Autodesk Fusion 360 part; units mm, degrees
note: some values were not read from the file. Set by a fixed rule: which face or edge a step refers to.
(part 4 of 5)
extrude "Extrude1''''''''''''" add sketch "Sketch1 (10)" along normal blind 5 separate body contours A14 L68 | A14 A15 A16 A17 L68 L69 L70 L71 | A15 L68 | A16 L70 | A17 L70 | L18 L19 L20 L21 picked at (89.8243, -16.6208) picked at (113.8243, -16.6208) picked at (90.3265, -30.2159) picked at (114.3265, -30.2159) makes body 18 in component "R_R_Wheel_Base"
sketch "Sketch2 (11)" plane through (0, -31.65, 0) normal (0, -1, 0) x (1, 0, 0) in component "R_R_Wheel_Base"
  circle A0 centre (115.415, -23.47) radius 1
  circle A1 centre (89.585, -23.47) radius 1
  line L0 (118, -30.47) -> (118, -16.47)
  line L1 (118, -16.47) -> (87, -16.47)
  line L2 (87, -16.47) -> (87, -30.47)
  line L3 (87, -30.47) -> (118, -30.47)
  line L4 (112, -28) -> (93, -28)
  line L5 (93, -28) -> (93, -18.94)
  line L6 (93, -18.94) -> (112, -18.94)
  line L7 (112, -18.94) -> (112, -28)
  line L8 (112, -28) -> (93, -18.94) construction
  line L9 (93, -28) -> (112, -18.94) construction
  point P0 (102.5, -23.47)
  constraint horizontal L4
  constraint perpendicular L4 L5
  constraint parallel L4 L6
  constraint parallel L5 L7
  constraint coincident L8 P0
  constraint coincident L9 P0
extrude "Extrude2''''''''''" add sketch "Sketch2 (11)" along normal blind 16 contours L4 L5 L6 L7 bodies 18 in component "R_R_Wheel_Base"
sketch "Sketch3 (7)" plane through (0, 0, -28) normal (0, 0, -1) x (-1, 0, 0) in component "R_R_Wheel_Base"
  line L0 (-93, -31.65) -> (-112, -31.65)
  line L1 (-112, -31.65) -> (-112, -47.65)
  line L2 (-112, -47.65) -> (-93, -47.65)
  line L3 (-93, -47.65) -> (-93, -31.65)
  line L4 (-93, -39.65) -> (-112, -47.65)
  line L5 (-93, -31.65) -> (-112, -39.65)
  line L6 (-112, -47.65) -> (-135.0409, -57.3514)
  line L7 (-135.0409, -57.3514) -> (-139.3591, -47.0957) construction
  line L8 (-112, -39.65) -> (-137.9021, -50.5561)
  line L9 (-150.0409, -57.3514) -> (-150.0409, -72.3514)
  line L10 (-150.0409, -72.3514) -> (-135.0409, -72.3514)
  line L11 (-135.0409, -72.3514) -> (-135.0409, -57.3514)
  line L12 (-150.0409, -57.3514) -> (-150.0409, -50.5561)
  line L13 (-150.0409, -50.5561) -> (-137.9021, -50.5561)
  line L14 (-135.0409, -57.3514) -> (-150.0409, -57.3514)
  dimension "d472" = 25
  dimension "d473" = 15
  dimension "d474" = 15
  dimension "d476" = 157.166
  dimension "d477" = 6.7953
  constraint midpoint L3 L4.start
  constraint coincident L1.end L2.start
  constraint coincident L0.start L3.end
  constraint midpoint L1 L5.end
  constraint parallel L4 L6
  constraint perpendicular L6 L7
  constraint coincident L7 L8.end
  constraint perpendicular L7 L8
  constraint vertical L9
  constraint horizontal L10
  constraint vertical L11
  constraint perpendicular L12 L13
  measures "d472" distance of L1.end L6.end
  measures "d473" distance of L6.end L9.start
  measures "d474" distance of L6.end L10.end
  measures "d476" angle of L8 L13
  measures "d477" distance of L9.start L12.end
extrude "Extrude4''''''''" add sketch "Sketch3 (7)" against normal blind 20 separate body contours L9 L10 L11 L14 makes body 19 in component "R_R_Wheel_Base"
extrude "Extrude3''''''''" add sketch "Sketch3 (7)" against normal blind 9.06 contours L1 L6 L8 L12 L13 L14 bodies 18 in component "R_R_Wheel_Base"
sketch "Sketch4 (9)" plane through (0, -26.65, 0) normal (0, 1, 0) x (-1, 0, 0) in component "R_R_Wheel_Base"
  circle A0 centre (-115.415, -23.47) radius 1
  circle A1 centre (-89.585, -23.47) radius 1
  line L0 (-118, -16.47) -> (-118, -30.47)
  line L1 (-118, -30.47) -> (-87, -30.47)
  line L2 (-87, -30.47) -> (-87, -16.47)
  line L3 (-87, -16.47) -> (-118, -16.47)
  line L4 (-112.5, -27.97) -> (-92.5, -27.97) construction
  line L5 (-92.5, -27.97) -> (-92.5, -18.97) construction
  line L6 (-92.5, -18.97) -> (-112.5, -18.97) construction
  line L7 (-92.5, -27.97) -> (-112.5, -27.97)
  line L8 (-112.5, -27.97) -> (-112.5, -18.97)
  line L9 (-112.5, -18.97) -> (-92.5, -18.97)
  line L10 (-92.5, -18.97) -> (-92.5, -27.97)
  line L11 (-112.41, -19.06) -> (-92.59, -19.06)
  line L12 (-92.59, -19.06) -> (-92.59, -27.88)
  line L13 (-92.59, -27.88) -> (-112.41, -27.88)
  line L14 (-112.41, -27.88) -> (-112.41, -19.06)
  dimension "d482" = 20
  dimension "d483" = 0.09
  constraint coincident L5.end L6.start
  constraint perpendicular L5 L6
  constraint horizontal L7
  constraint vertical L8
  constraint horizontal L9
  constraint vertical L10
  constraint coincident L4.end L5.start
  measures "d482" distance of L5.end L6.end
extrude "Extrude5'''''" add sketch "Sketch4 (9)" along normal blind 3 contours L11 L12 L13 L14 bodies 18 in component "R_R_Wheel_Base"
sketch "Sketch5 (6)" plane through (0, 0, -28) normal (0, 0, -1) x (-1, 0, 0) in component "R_R_Wheel_Base"
  line L0 (-135.0409, -57.3514) -> (-150.0409, -57.3514)
  line L1 (-150.0409, -57.3514) -> (-150.0409, -72.3514)
  line L2 (-150.0409, -72.3514) -> (-135.0409, -72.3514)
  line L3 (-135.0409, -72.3514) -> (-135.0409, -57.3514)
  line L4 (-136.4409, -69.9514) -> (-148.6409, -69.9514)
  line L5 (-148.6409, -69.9514) -> (-148.6409, -59.7514)
  line L6 (-148.6409, -59.7514) -> (-136.4409, -59.7514)
  line L7 (-136.4409, -59.7514) -> (-136.4409, -69.9514)
  line L8 (-136.4409, -69.9514) -> (-148.6409, -59.7514) construction
  line L9 (-148.6409, -69.9514) -> (-136.4409, -59.7514) construction
  point P0 (-142.5409, -64.8514)
  dimension "d486" = 12.2
  dimension "d487" = 10.2
  constraint horizontal L4
  constraint perpendicular L4 L5
  constraint parallel L4 L6
  constraint parallel L5 L7
  constraint coincident L8 P0
  constraint coincident L9 P0
  measures "d486" distance of L5.end L6.end
  measures "d487" distance of L4.end L5.end
extrude "Extrude6'''''" cut sketch "Sketch5 (6)" against normal blind 18.841 contours L4 L5 L6 L7 bodies 19 in component "R_R_Wheel_Base"
sketch "Sketch6 (6)" plane through (0, 0, -8) normal (0, 0, 1) x (1, 0, 0) in component "R_R_Wheel_Base"
  line L0 (150.0409, -57.3514) -> (135.0409, -57.3514)
  line L1 (135.0409, -57.3514) -> (135.0409, -72.3514)
  line L2 (135.0409, -72.3514) -> (150.0409, -72.3514)
  line L3 (150.0409, -72.3514) -> (150.0409, -57.3514)
  circle A0 centre (142.5409, -64.8514) radius 2
  dimension "d490" = 4
  measures "d490" diameter of A0
extrude "Extrude7''" cut sketch "Sketch6 (6)" against normal blind 1.159 contours A0 bodies 19 in component "R_R_Wheel_Base"
sketch "Sketch7 (4)" plane through (0, 0, -8) normal (0, 0, 1) x (1, 0, 0) in component "R_R_Wheel_Base"
  circle A0 centre (142.5409, -64.8514) radius 2
  line L0 (150.0409, -57.3514) -> (135.0409, -57.3514)
  line L1 (135.0409, -57.3514) -> (135.0409, -72.3514)
  line L2 (135.0409, -72.3514) -> (150.0409, -72.3514)
  line L3 (150.0409, -72.3514) -> (150.0409, -57.3514)
  line L4 (142.5409, -64.8514) -> (137.9689, -64.8514) construction
  line L5 (142.5409, -64.8514) -> (147.1129, -64.8514) construction
  circle A1 centre (137.9689, -64.8514) radius 0.75
  circle A2 centre (147.1129, -64.8514) radius 0.75
  dimension "d493" = 4.572
  dimension "d494" = 4.572
  dimension "d495" = 1.5
  dimension "d496" = 1.5
  constraint coincident A0.centre L4.start
  constraint horizontal L4
  constraint parallel L4 L5
  constraint coincident L4.end A1.centre
  constraint coincident L5.end A2.centre
  measures "d493" distance of A0.centre L4.end
  measures "d494" distance of A0.centre L5.end
  measures "d495" diameter of A1
  measures "d496" diameter of A2
extrude "Extrude8''" cut sketch "Sketch7 (4)" against normal blind 1.159 contours A1 | A2 bodies 19 in component "R_R_Wheel_Base"
sketch "Sketch1 (11)" plane through (0, -26.65, 0) normal (0, -1, 0) x (1, 0, 0) in component "L_R_Wheel_Base"
  line L0 (0, -40) -> (-5, -45)
  line L1 (-5, -45) -> (-5, -79.85)
  line L2 (-5, -79.85) -> (0, -84.85)
  line L3 (0, -84.85) -> (0, -97)
  arc A0 (0, -97) -> (3, -100) centre (3, -97) ccw
  line L4 (3, -100) -> (6, -103)
  line L5 (6, -103) -> (25, -103)
  line L6 (25, -103) -> (28, -100)
  line L7 (28, -100) -> (154, -100)
  arc A1 (154, -100) -> (157, -97) centre (154, -97) ccw
  line L8 (157, -97) -> (157, -94)
  arc A2 (160, -91) -> (157, -94) centre (160, -94) ccw
  line L9 (160, -91) -> (181.27, -91)
  arc A3 (181.27, -91) -> (184.27, -88) centre (181.27, -88) ccw
  line L10 (184.27, -88) -> (184.27, -12)
  arc A4 (184.27, -12) -> (181.27, -9) centre (181.27, -12) ccw
  line L11 (181.27, -9) -> (160, -9)
  arc A5 (157, -6) -> (160, -9) centre (160, -6) ccw
  line L12 (157, -6) -> (157, -3)
  arc A6 (157, -3) -> (154, 0) centre (154, -3) ccw
  line L13 (154, 0) -> (28, 0)
  line L14 (28, 0) -> (25, 3)
  line L15 (25, 3) -> (6, 3)
  line L16 (6, 3) -> (3, 0)
  arc A7 (3, 0) -> (0, -3) centre (3, -3) ccw
  line L17 (0, -3) -> (0, -40)
  circle A8 centre (3, -97) radius 1.0625
  circle A9 centre (3, -71) radius 1.0625
  circle A10 centre (22, -71) radius 1.0625
  circle A11 centre (3, -29) radius 1.0625
  circle A12 centre (3, -3) radius 1.0625
  circle A13 centre (22, -29) radius 1.0625
  circle A14 centre (90, -16) radius 1.0625
  circle A15 centre (114, -16) radius 1.0625
  circle A16 centre (90, -30.28) radius 1.0625
  circle A17 centre (114, -30.28) radius 1.0625
  circle A18 centre (114, -69.72) radius 1.0625
  circle A19 centre (90, -84) radius 1.0625
  circle A20 centre (90, -69.72) radius 1.0625
  circle A21 centre (114, -84) radius 1.0625
  line L18 (92.5, -27.97) -> (92.5, -18.97)
  line L19 (92.5, -18.97) -> (112.5, -18.97)
  line L20 (112.5, -18.97) -> (112.5, -27.97)
  line L21 (112.5, -27.97) -> (92.5, -27.97)
  circle A22 centre (11.5, -70.07) radius 1
  circle A23 centre (11.5, -4.1) radius 1
  circle A24 centre (11.5, -29.93) radius 1
  line L22 (92.5, -81.36) -> (92.5, -72.36)
  line L23 (92.5, -72.36) -> (112.5, -72.36)
  line L24 (112.5, -72.36) -> (112.5, -81.36)
  line L25 (112.5, -81.36) -> (92.5, -81.36)
  circle A25 centre (89.585, -23.47) radius 1
  circle A26 centre (115.415, -76.86) radius 1
  line L26 (16, -72.97) -> (16, -93)
  line L27 (16, -93) -> (7, -93)
  line L28 (7, -93) -> (7, -72.97)
  line L29 (7, -72.97) -> (16, -72.97)
  line L30 (16, -7) -> (16, -27.03)
  line L31 (16, -27.03) -> (7, -27.03)
  line L32 (7, -27.03) -> (7, -7)
  line L33 (7, -7) -> (16, -7)
  circle A27 centre (11.5, -95.9) radius 1
  circle A28 centre (89.585, -76.86) radius 1
  circle A29 centre (115.415, -23.47) radius 1
  line L34 (127.5, -73.5) -> (124.5, -73.5)
  line L35 (124.5, -73.5) -> (124.5, -68.5)
  line L36 (124.5, -68.5) -> (127.5, -68.5)
  line L37 (127.5, -68.5) -> (127.5, -73.5)
  line L38 (183.5, -73.5) -> (180.5, -73.5)
  line L39 (180.5, -73.5) -> (180.5, -68.5)
  line L40 (180.5, -68.5) -> (183.5, -68.5)
  line L41 (183.5, -68.5) -> (183.5, -73.5)
  line L42 (127.5, -31.5) -> (124.5, -31.5)
  line L43 (124.5, -31.5) -> (124.5, -26.5)
  line L44 (124.5, -26.5) -> (127.5, -26.5)
  line L45 (127.5, -26.5) -> (127.5, -31.5)
  line L46 (183.5, -31.5) -> (180.5, -31.5)
  line L47 (180.5, -31.5) -> (180.5, -26.5)
  line L48 (180.5, -26.5) -> (183.5, -26.5)
  line L49 (183.5, -26.5) -> (183.5, -31.5)
  line L50 (36.83, -3.81) -> (36.83, -13.97)
  line L51 (36.83, -13.97) -> (19.05, -13.97)
  line L52 (19.05, -13.97) -> (19.05, -3.81)
  line L53 (19.05, -3.81) -> (36.83, -3.81)
  line L54 (36.83, -96.52) -> (19.05, -96.52)
  line L55 (19.05, -96.52) -> (19.05, -86.36)
  line L56 (19.05, -86.36) -> (36.83, -86.36)
  line L57 (36.83, -86.36) -> (36.83, -96.52)
  line L58 (114.3, -3.81) -> (130.81, -3.81)
  line L59 (130.81, -3.81) -> (130.81, -13.97)
  line L60 (130.81, -13.97) -> (114.3, -13.97)
  line L61 (114.3, -13.97) -> (114.3, -3.81)
  line L62 (114.3, -96.52) -> (114.3, -86.36)
  line L63 (114.3, -86.36) -> (130.81, -86.36)
  line L64 (130.81, -86.36) -> (130.81, -96.52)
  line L65 (130.81, -96.52) -> (114.3, -96.52)
  line L66 (89.585, -23.47) -> (115.415, -23.47) construction
  line L67 (102.5, -23.47) -> (102.5, -29.6509) construction
  line L68 (118, -16.47) -> (87, -16.47)
  line L69 (87, -16.47) -> (87, -30.47)
  line L70 (87, -30.47) -> (118, -30.47)
  line L71 (118, -30.47) -> (118, -16.47)
  line L72 (118, -16.47) -> (87, -30.47) construction
  line L73 (87, -16.47) -> (118, -30.47) construction
  point P0 (102.5, -23.47)
  dimension "d466_1" = 31
  dimension "d467_1" = 14
  constraint coincident A25.centre L66.start
  constraint coincident A29.centre L66.end
  constraint midpoint L66 P0
  constraint perpendicular L66 L67
  constraint horizontal L68
  constraint perpendicular L68 L69
  constraint parallel L68 L70
  constraint parallel L69 L71
  constraint coincident L72 P0
  constraint coincident L73 P0
  constraint coincident P0 L67.start
  measures "d466_1" distance of L69.end L70.end
  measures "d467_1" distance of L68.end L69.end
extrude "Extrude1'''''''''''''" add sketch "Sketch1 (11)" along normal blind 5 separate body contours A14 L68 | A14 A15 A16 A17 L68 L69 L70 L71 | A15 L68 | A16 L70 | A17 L70 | L18 L19 L20 L21 picked at (89.8243, -16.6208) picked at (113.8243, -16.6208) picked at (90.3265, -30.2159) picked at (114.3265, -30.2159) makes body 20 in component "L_R_Wheel_Base"
sketch "Sketch2 (12)" plane through (0, -31.65, 0) normal (0, -1, 0) x (1, 0, 0) in component "L_R_Wheel_Base"
  circle A0 centre (115.415, -23.47) radius 1
  circle A1 centre (89.585, -23.47) radius 1
  line L0 (118, -30.47) -> (118, -16.47)
  line L1 (118, -16.47) -> (87, -16.47)
  line L2 (87, -16.47) -> (87, -30.47)
  line L3 (87, -30.47) -> (118, -30.47)
  line L4 (112, -28) -> (93, -28)
  line L5 (93, -28) -> (93, -18.94)
  line L6 (93, -18.94) -> (112, -18.94)
  line L7 (112, -18.94) -> (112, -28)
  line L8 (112, -28) -> (93, -18.94) construction
  line L9 (93, -28) -> (112, -18.94) construction
  point P0 (102.5, -23.47)
  constraint horizontal L4
  constraint perpendicular L4 L5
  constraint parallel L4 L6
  constraint parallel L5 L7
  constraint coincident L8 P0
  constraint coincident L9 P0
extrude "Extrude2'''''''''''" add sketch "Sketch2 (12)" along normal blind 16 contours L4 L5 L6 L7 bodies 20 in component "L_R_Wheel_Base"
sketch "Sketch3 (8)" plane through (0, 0, -28) normal (0, 0, -1) x (-1, 0, 0) in component "L_R_Wheel_Base"
  line L0 (-93, -31.65) -> (-112, -31.65)
  line L1 (-112, -31.65) -> (-112, -47.65)
  line L2 (-112, -47.65) -> (-93, -47.65)
  line L3 (-93, -47.65) -> (-93, -31.65)
  line L4 (-93, -39.65) -> (-112, -47.65)
  line L5 (-93, -31.65) -> (-112, -39.65)
  line L6 (-112, -47.65) -> (-135.0409, -57.3514)
  line L7 (-135.0409, -57.3514) -> (-139.3591, -47.0957) construction
  line L8 (-112, -39.65) -> (-137.9021, -50.5561)
  line L9 (-150.0409, -57.3514) -> (-150.0409, -72.3514)
  line L10 (-150.0409, -72.3514) -> (-135.0409, -72.3514)
  line L11 (-135.0409, -72.3514) -> (-135.0409, -57.3514)
  line L12 (-150.0409, -57.3514) -> (-150.0409, -50.5561)
  line L13 (-150.0409, -50.5561) -> (-137.9021, -50.5561)
  line L14 (-135.0409, -57.3514) -> (-150.0409, -57.3514)
  dimension "d472_1" = 25
  dimension "d473_1" = 15
  dimension "d474_1" = 15
  dimension "d476_1" = 157.166
  dimension "d477_1" = 6.7953
  constraint midpoint L3 L4.start
  constraint coincident L1.end L2.start
  constraint coincident L0.start L3.end
  constraint midpoint L1 L5.end
  constraint parallel L4 L6
  constraint perpendicular L6 L7
  constraint coincident L7 L8.end
  constraint perpendicular L7 L8
  constraint vertical L9
  constraint horizontal L10
  constraint vertical L11
  constraint perpendicular L12 L13
  measures "d472_1" distance of L1.end L6.end
  measures "d473_1" distance of L6.end L9.start
  measures "d474_1" distance of L6.end L10.end
  measures "d476_1" angle of L8 L13
  measures "d477_1" distance of L9.start L12.end
extrude "Extrude4'''''''''" add sketch "Sketch3 (8)" against normal blind 20 separate body contours L9 L10 L11 L14 makes body 21 in component "L_R_Wheel_Base"
extrude "Extrude3'''''''''" add sketch "Sketch3 (8)" against normal blind 9.06 contours L1 L6 L8 L12 L13 L14 bodies 20 in component "L_R_Wheel_Base"
sketch "Sketch4 (10)" plane through (0, -26.65, 0) normal (0, 1, 0) x (-1, 0, 0) in component "L_R_Wheel_Base"
  circle A0 centre (-115.415, -23.47) radius 1
  circle A1 centre (-89.585, -23.47) radius 1
  line L0 (-118, -16.47) -> (-118, -30.47)
  line L1 (-118, -30.47) -> (-87, -30.47)
  line L2 (-87, -30.47) -> (-87, -16.47)
  line L3 (-87, -16.47) -> (-118, -16.47)
  line L4 (-112.5, -27.97) -> (-92.5, -27.97) construction
  line L5 (-92.5, -27.97) -> (-92.5, -18.97) construction
  line L6 (-92.5, -18.97) -> (-112.5, -18.97) construction
  line L7 (-92.5, -27.97) -> (-112.5, -27.97)
  line L8 (-112.5, -27.97) -> (-112.5, -18.97)
  line L9 (-112.5, -18.97) -> (-92.5, -18.97)
  line L10 (-92.5, -18.97) -> (-92.5, -27.97)
  line L11 (-112.41, -19.06) -> (-92.59, -19.06)
  line L12 (-92.59, -19.06) -> (-92.59, -27.88)
  line L13 (-92.59, -27.88) -> (-112.41, -27.88)
  line L14 (-112.41, -27.88) -> (-112.41, -19.06)
  dimension "d482_1" = 20
  dimension "d483_1" = 0.09
  constraint coincident L5.end L6.start
  constraint perpendicular L5 L6
  constraint horizontal L7
  constraint vertical L8
  constraint horizontal L9
  constraint vertical L10
  constraint coincident L4.end L5.start
  measures "d482_1" distance of L5.end L6.end
extrude "Extrude5''''''" add sketch "Sketch4 (10)" along normal blind 3 contours L11 L12 L13 L14 bodies 20 in component "L_R_Wheel_Base"
sketch "Sketch5 (7)" plane through (0, 0, -28) normal (0, 0, -1) x (-1, 0, 0) in component "L_R_Wheel_Base"
  line L0 (-135.0409, -57.3514) -> (-150.0409, -57.3514)
  line L1 (-150.0409, -57.3514) -> (-150.0409, -72.3514)
  line L2 (-150.0409, -72.3514) -> (-135.0409, -72.3514)
  line L3 (-135.0409, -72.3514) -> (-135.0409, -57.3514)
  line L4 (-136.4409, -69.9514) -> (-148.6409, -69.9514)
  line L5 (-148.6409, -69.9514) -> (-148.6409, -59.7514)
  line L6 (-148.6409, -59.7514) -> (-136.4409, -59.7514)
  line L7 (-136.4409, -59.7514) -> (-136.4409, -69.9514)
  line L8 (-136.4409, -69.9514) -> (-148.6409, -59.7514) construction
  line L9 (-148.6409, -69.9514) -> (-136.4409, -59.7514) construction
  point P0 (-142.5409, -64.8514)
  dimension "d486_1" = 12.2
  dimension "d487_1" = 10.2
  constraint horizontal L4
  constraint perpendicular L4 L5
  constraint parallel L4 L6
  constraint parallel L5 L7
  constraint coincident L8 P0
  constraint coincident L9 P0
  measures "d486_1" distance of L5.end L6.end
  measures "d487_1" distance of L4.end L5.end
extrude "Extrude6''''''" cut sketch "Sketch5 (7)" against normal blind 18.841 contours L4 L5 L6 L7 bodies 21 in component "L_R_Wheel_Base"
sketch "Sketch6 (7)" plane through (0, 0, -8) normal (0, 0, 1) x (1, 0, 0) in component "L_R_Wheel_Base"
  line L0 (150.0409, -57.3514) -> (135.0409, -57.3514)
  line L1 (135.0409, -57.3514) -> (135.0409, -72.3514)
  line L2 (135.0409, -72.3514) -> (150.0409, -72.3514)
  line L3 (150.0409, -72.3514) -> (150.0409, -57.3514)
  circle A0 centre (142.5409, -64.8514) radius 2
  dimension "d490_1" = 4
  measures "d490_1" diameter of A0
extrude "Extrude7'''" cut sketch "Sketch6 (7)" against normal blind 1.159 contours A0 bodies 21 in component "L_R_Wheel_Base"
sketch "Sketch7 (5)" plane through (0, 0, -8) normal (0, 0, 1) x (1, 0, 0) in component "L_R_Wheel_Base"
  circle A0 centre (142.5409, -64.8514) radius 2
  line L0 (150.0409, -57.3514) -> (135.0409, -57.3514)
  line L1 (135.0409, -57.3514) -> (135.0409, -72.3514)
  line L2 (135.0409, -72.3514) -> (150.0409, -72.3514)
  line L3 (150.0409, -72.3514) -> (150.0409, -57.3514)
  line L4 (142.5409, -64.8514) -> (137.9689, -64.8514) construction
  line L5 (142.5409, -64.8514) -> (147.1129, -64.8514) construction
  circle A1 centre (137.9689, -64.8514) radius 0.75
  circle A2 centre (147.1129, -64.8514) radius 0.75
  dimension "d493_1" = 4.572
  dimension "d494_1" = 4.572
  dimension "d495_1" = 1.5
  dimension "d496_1" = 1.5
  constraint coincident A0.centre L4.start
  constraint horizontal L4
  constraint parallel L4 L5
  constraint coincident L4.end A1.centre
  constraint coincident L5.end A2.centre
  measures "d493_1" distance of A0.centre L4.end
  measures "d494_1" distance of A0.centre L5.end
  measures "d495_1" diameter of A1
  measures "d496_1" diameter of A2
extrude "Extrude8'''" cut sketch "Sketch7 (5)" against normal blind 1.159 contours A1 | A2 bodies 21 in component "L_R_Wheel_Base"
fillet "Fillet1'''" radius 7 3 edges at (112, -39.65, -23.47) (137.9021, -50.5561, -23.47) (150.0409, -50.5561, -23.47) on bodies 18 in component "R_R_Wheel_Base"
fillet "Fillet2''''" radius 14 1 edges at (93, -47.65, -23.47) on bodies 18 in component "R_R_Wheel_Base"
extrude "Extrude9''" add 1 faces at (140.5076, -59.7514, -21.7197) along direction (0, -1, 0) blind 10.2 on bodies 21 bodies 21 in component "L_R_Wheel_Base"
extrude "Extrude10'" add 1 faces at (145.0409, -62.3514, -28) along direction (0, 0, -1) blind 10.94 on bodies 21 bodies 21 20 in component "L_R_Wheel_Base"
extrude "Extrude11'" cut 1 faces at (142.5907, -59.1866, -8) along direction (0, 0, -1) blind 10.94 on bodies 21 bodies 21 in component "L_R_Wheel_Base"
extrude "Extrude12'" cut 3 faces at (142.6632, -65.4169, -9.159) (146.8923, -64.6814, -9.159) (137.6381, -65.1805, -9.159) along direction (0, 0, -1) blind 29.781 on bodies 21 bodies 21 in component "L_R_Wheel_Base"
sketch "Sketch8 (2)" plane through (0, 0, -18.94) normal (0, 0, 1) x (1, 0, 0) in component "L_R_Wheel_Base"
  circle A0 centre (142.5409, -64.8514) radius 2
  circle A1 centre (137.9689, -64.8514) radius 0.75
  circle A2 centre (147.1129, -64.8514) radius 0.75
  line L0 (112, -31.65) -> (93, -31.65)
  line L1 (93, -31.65) -> (93, -47.65)
  line L2 (93, -47.65) -> (112, -47.65)
  line L3 (112, -47.65) -> (135.0409, -57.3514)
  line L4 (135.0409, -57.3514) -> (135.0409, -72.3514)
  line L5 (135.0409, -72.3514) -> (150.0409, -72.3514)
  line L6 (150.0409, -72.3514) -> (150.0409, -50.5561)
  line L7 (150.0409, -50.5561) -> (137.9021, -50.5561)
  line L8 (137.9021, -50.5561) -> (112, -39.65)
  line L9 (112, -39.65) -> (112, -31.65)
  line L10 (148.6409, -69.9514) -> (136.4409, -69.9514)
  line L11 (136.4409, -69.9514) -> (136.4409, -59.7514)
  line L12 (136.4409, -59.7514) -> (148.6409, -59.7514)
  line L13 (148.6409, -59.7514) -> (148.6409, -69.9514)
  line L14 (148.6409, -69.9514) -> (136.4409, -59.7514) construction
  line L15 (136.4409, -69.9514) -> (148.6409, -59.7514) construction
  point P0 (142.5409, -64.8514)
  dimension "d510" = 12.2
  dimension "d511" = 10.2
  constraint horizontal L10
  constraint perpendicular L10 L11
  constraint parallel L10 L12
  constraint parallel L11 L13
  constraint coincident L14 P0
  constraint coincident L15 P0
  constraint coincident P0 A0.centre
  measures "d510" distance of L11.end L12.end
  measures "d511" distance of L10.end L11.end
extrude "Extrude13''" cut sketch "Sketch8 (2)" against normal blind 18.841 contours A0 | A1 | A2 | L10 L11 L12 L13 bodies 21 in component "L_R_Wheel_Base"
fillet "Fillet1''''" radius 7 3 edges at (112, -39.65, -23.47) (137.9021, -50.5561, -23.47) (150.0409, -50.5561, -23.47) on bodies 21 in component "L_R_Wheel_Base"
fillet "Fillet2'''''" radius 14 1 edges at (93, -47.65, -23.47) on bodies 21 in component "L_R_Wheel_Base"
combine "Combine1" operation add target body 18 tool bodies 19 in component "R_R_Wheel_Base"
sketch "Sketch1 (12)" plane through (0, -26.65, 0) normal (0, -1, 0) x (1, 0, 0) in component "R_F_Wheel_Base"
  line L0 (0, -40) -> (-5, -45)
  line L1 (-5, -45) -> (-5, -79.85)
  line L2 (-5, -79.85) -> (0, -84.85)
  line L3 (0, -84.85) -> (0, -97)
  arc A0 (0, -97) -> (3, -100) centre (3, -97) ccw
  line L4 (3, -100) -> (6, -103)
  line L5 (6, -103) -> (25, -103)
  line L6 (25, -103) -> (28, -100)
  line L7 (28, -100) -> (154, -100)
  arc A1 (154, -100) -> (157, -97) centre (154, -97) ccw
  line L8 (157, -97) -> (157, -94)
  arc A2 (160, -91) -> (157, -94) centre (160, -94) ccw
  line L9 (160, -91) -> (181.27, -91)
  arc A3 (181.27, -91) -> (184.27, -88) centre (181.27, -88) ccw
  line L10 (184.27, -88) -> (184.27, -12)
  arc A4 (184.27, -12) -> (181.27, -9) centre (181.27, -12) ccw
  line L11 (181.27, -9) -> (160, -9)
  arc A5 (157, -6) -> (160, -9) centre (160, -6) ccw
  line L12 (157, -6) -> (157, -3)
  arc A6 (157, -3) -> (154, 0) centre (154, -3) ccw
  line L13 (154, 0) -> (28, 0)
  line L14 (28, 0) -> (25, 3)
  line L15 (25, 3) -> (6, 3)
  line L16 (6, 3) -> (3, 0)
  arc A7 (3, 0) -> (0, -3) centre (3, -3) ccw
  line L17 (0, -3) -> (0, -40)
  circle A8 centre (3, -97) radius 1.0625
  circle A9 centre (3, -71) radius 1.0625
  circle A10 centre (22, -71) radius 1.0625
  circle A11 centre (3, -29) radius 1.0625
  circle A12 centre (3, -3) radius 1.0625
  circle A13 centre (22, -29) radius 1.0625
  circle A14 centre (90, -16) radius 1.0625
  circle A15 centre (114, -16) radius 1.0625
  circle A16 centre (90, -30.28) radius 1.0625
  circle A17 centre (114, -30.28) radius 1.0625
  circle A18 centre (114, -69.72) radius 1.0625
  circle A19 centre (90, -84) radius 1.0625
  circle A20 centre (90, -69.72) radius 1.0625
  circle A21 centre (114, -84) radius 1.0625
  line L18 (92.5, -27.97) -> (92.5, -18.97)
  line L19 (92.5, -18.97) -> (112.5, -18.97)
  line L20 (112.5, -18.97) -> (112.5, -27.97)
  line L21 (112.5, -27.97) -> (92.5, -27.97)
  circle A22 centre (11.5, -70.07) radius 1
  circle A23 centre (11.5, -4.1) radius 1
  circle A24 centre (11.5, -29.93) radius 1
  line L22 (92.5, -81.36) -> (92.5, -72.36)
  line L23 (92.5, -72.36) -> (112.5, -72.36)
  line L24 (112.5, -72.36) -> (112.5, -81.36)
  line L25 (112.5, -81.36) -> (92.5, -81.36)
  circle A25 centre (89.585, -23.47) radius 1
  circle A26 centre (115.415, -76.86) radius 1
  line L26 (16, -72.97) -> (16, -93)
  line L27 (16, -93) -> (7, -93)
  line L28 (7, -93) -> (7, -72.97)
  line L29 (7, -72.97) -> (16, -72.97)
  line L30 (16, -7) -> (16, -27.03)
  line L31 (16, -27.03) -> (7, -27.03)
  line L32 (7, -27.03) -> (7, -7)
  line L33 (7, -7) -> (16, -7)
  circle A27 centre (11.5, -95.9) radius 1
  circle A28 centre (89.585, -76.86) radius 1
  circle A29 centre (115.415, -23.47) radius 1
  line L34 (127.5, -73.5) -> (124.5, -73.5)
  line L35 (124.5, -73.5) -> (124.5, -68.5)
  line L36 (124.5, -68.5) -> (127.5, -68.5)
  line L37 (127.5, -68.5) -> (127.5, -73.5)
  line L38 (183.5, -73.5) -> (180.5, -73.5)
  line L39 (180.5, -73.5) -> (180.5, -68.5)
  line L40 (180.5, -68.5) -> (183.5, -68.5)
  line L41 (183.5, -68.5) -> (183.5, -73.5)
  line L42 (127.5, -31.5) -> (124.5, -31.5)
  line L43 (124.5, -31.5) -> (124.5, -26.5)
  line L44 (124.5, -26.5) -> (127.5, -26.5)
  line L45 (127.5, -26.5) -> (127.5, -31.5)
  line L46 (183.5, -31.5) -> (180.5, -31.5)
  line L47 (180.5, -31.5) -> (180.5, -26.5)
  line L48 (180.5, -26.5) -> (183.5, -26.5)
  line L49 (183.5, -26.5) -> (183.5, -31.5)
  line L50 (36.83, -3.81) -> (36.83, -13.97)
  line L51 (36.83, -13.97) -> (19.05, -13.97)
  line L52 (19.05, -13.97) -> (19.05, -3.81)
  line L53 (19.05, -3.81) -> (36.83, -3.81)
  line L54 (36.83, -96.52) -> (19.05, -96.52)
  line L55 (19.05, -96.52) -> (19.05, -86.36)
  line L56 (19.05, -86.36) -> (36.83, -86.36)
  line L57 (36.83, -86.36) -> (36.83, -96.52)
  line L58 (114.3, -3.81) -> (130.81, -3.81)
  line L59 (130.81, -3.81) -> (130.81, -13.97)
  line L60 (130.81, -13.97) -> (114.3, -13.97)
  line L61 (114.3, -13.97) -> (114.3, -3.81)
  line L62 (114.3, -96.52) -> (114.3, -86.36)
  line L63 (114.3, -86.36) -> (130.81, -86.36)
  line L64 (130.81, -86.36) -> (130.81, -96.52)
  line L65 (130.81, -96.52) -> (114.3, -96.52)
  line L66 (5.5, -5.015) -> (5.5, -29.015)
  line L67 (17.5, -29.015) -> (17.5, -5.015)
  line L68 (17.5, -5.015) -> (5.5, -29.015) construction
  line L69 (5.5, -5.015) -> (17.5, -29.015) construction
  line L70 (7, -3) -> (7, -5.015) construction
  line L71 (16, -3) -> (16, -5.015) construction
  line L72 (7.1, -3) -> (7.1, -5.015) construction
  line L73 (15.9, -3) -> (15.9, -5.015) construction
  line L74 (5.5, -5.015) -> (7.1, -5.015)
  line L75 (17.5, -5.015) -> (15.9, -5.015)
  line L76 (15.9, -5.015) -> (15.9, -0.5642)
  line L77 (15.9, -0.5642) -> (7.1, -0.5642)
  line L78 (7.1, -0.5642) -> (7.1, -5.015)
  line L79 (5.5, -29.015) -> (7.1, -29.015)
  line L80 (17.5, -29.015) -> (15.9, -29.015)
  line L81 (7.1, -29.015) -> (7.1, -33.466)
  line L82 (7.1, -33.466) -> (15.9, -33.466)
  line L83 (15.9, -33.466) -> (15.9, -29.015)
  point P0 (11.5, -17.015)
  dimension "d517" = 12
  dimension "d518" = 24
  dimension "d519" = -0.1
  dimension "d520" = 0.1
  dimension "d521" = 1.6
  dimension "d522" = 4.4508
  dimension "d523" = 8.8
  dimension "d524" = 4.4508
  dimension "d525" = 1.6
  dimension "d526" = 3.5642
  dimension "d527" = 5.5
  dimension "d528" = 1.55
  dimension "d529" = 1.6
  dimension "d530" = 1.6
  dimension "d531" = 4.451
  dimension "d532" = 7.1
  dimension "d533" = 4.451
  dimension "d534" = 32.9018
  constraint parallel L66 L67
  constraint coincident L68 P0
  constraint coincident L69 P0
  constraint perpendicular L72 L74
  constraint perpendicular L73 L75
  constraint vertical L76
  constraint horizontal L77
  constraint vertical L78
  constraint perpendicular L17 L79
  constraint perpendicular L67 L80
  constraint vertical L81
  constraint horizontal L82
  constraint vertical L83
  measures "d517" distance of L66.end L67.start
  measures "d518" distance of L66.start L66.end
  measures "d521" distance of L67.end L73.end
  measures "d522" distance of L73.end L76.end
  measures "d523" distance of L76.end L77.end
  measures "d524" distance of L72.end L77.end
  measures "d525" distance of L66.start L72.end
  measures "d526" distance of L15 L77
  measures "d527" distance of L17 L66
  measures "d528" distance of L52 L67
  measures "d529" distance of L66.end L79.end
  measures "d530" distance of L67.start L80.end
  measures "d531" distance of L80.end L82.end
  measures "d532" distance of L17 L81
  measures "d533" distance of L79 L82
  measures "d534" distance of L77 L82
extrude "Extrude1''''''''''''''" add sketch "Sketch1 (12)" along normal blind 5 separate body contours L30 L31 L32 L33 | L66 L67 L74 L75 L76 L77 L78 L79 L80 L81 L82 L83 makes body 22 in component "R_F_Wheel_Base"
sketch "Sketch2 (13)" plane through (0, -31.65, 0) normal (0, -1, 0) x (1, 0, 0) in component "R_F_Wheel_Base"
  circle A0 centre (11.5, -4.1) radius 1
  circle A1 centre (11.5, -29.93) radius 1
  line L0 (5.5, -5.015) -> (5.5, -29.015)
  line L1 (5.5, -29.015) -> (7.1, -29.015)
  line L2 (7.1, -29.015) -> (7.1, -33.466)
  line L3 (7.1, -33.466) -> (15.9, -33.466)
  line L4 (15.9, -33.466) -> (15.9, -29.015)
  line L5 (15.9, -29.015) -> (17.5, -29.015)
  line L6 (17.5, -29.015) -> (17.5, -5.015)
  line L7 (17.5, -5.015) -> (15.9, -5.015)
  line L8 (15.9, -5.015) -> (15.9, -0.5642)
  line L9 (15.9, -0.5642) -> (7.1, -0.5642)
  line L10 (7.1, -0.5642) -> (7.1, -5.015)
  line L11 (7.1, -5.015) -> (5.5, -5.015)
  line L12 (16, -26.015) -> (7, -26.015)
  line L13 (7, -26.015) -> (7, -8.015)
  line L14 (7, -8.015) -> (16, -8.015)
  line L15 (16, -8.015) -> (16, -26.015)
  line L16 (16, -26.015) -> (7, -8.015) construction
  line L17 (7, -26.015) -> (16, -8.015) construction
  point P0 (11.5, -17.015)
  dimension "d537" = 18
  constraint horizontal L12
  constraint perpendicular L12 L13
  constraint parallel L12 L14
  constraint parallel L13 L15
  constraint coincident L16 P0
  constraint coincident L17 P0
  measures "d537" distance of L12.end L13.end
extrude "Extrude2''''''''''''" add sketch "Sketch2 (13)" along normal blind 16 contours L12 L13 L14 L15 bodies 22 in component "R_F_Wheel_Base"
sketch "Sketch3 (9)" plane through (0, 0, -26.015) normal (0, 0, -1) x (-1, 0, 0) in component "R_F_Wheel_Base"
  line L0 (-7, -31.65) -> (-16, -31.65)
  line L1 (-16, -31.65) -> (-16, -47.65)
  line L2 (-16, -47.65) -> (-7, -47.65)
  line L3 (-7, -47.65) -> (-7, -31.65)
  line L4 (-16, -39.65) -> (-7, -47.65)
  line L5 (-16, -31.65) -> (-7, -39.65)
  line L6 (-16, -47.65) -> (-16, -72.351) construction
  line L7 (-16, -72.351) -> (35, -72.351) construction
  line L8 (9.5, -72.351) -> (-5.5, -72.351)
  line L9 (-5.5, -72.351) -> (-5.5, -57.351)
  line L10 (9.5, -57.351) -> (9.5, -72.351)
  line L11 (9.5, -57.351) -> (1.25, -48.5005)
  line L12 (-7, -39.65) -> (1.25, -48.5005)
  line L13 (-7, -47.65) -> (-5.5, -57.351)
  dimension "d540" = 24.701
  dimension "d541" = 15
  dimension "d542" = 15
  constraint midpoint L1 L4.start
  constraint coincident L2.end L3.start
  constraint coincident L0.end L1.start
  constraint midpoint L3 L5.end
  constraint coincident L1.end L2.start
  constraint perpendicular L2 L6
  constraint perpendicular L6 L7
  constraint horizontal L8
  constraint vertical L9
  constraint vertical L10
  constraint midpoint L7 L8.start
  constraint parallel L11 L12
  measures "d540" distance of L1.end L6.end
  measures "d541" distance of L8.start L8.end
  measures "d542" distance of L8.start L10.start
extrude "Extrude3''''''''''" add sketch "Sketch3 (9)" against normal blind 20 contours L3 L8 L9 L10 L11 L12 L13 bodies 22 in component "R_F_Wheel_Base"
sketch "Sketch4 (11)" plane through (0, 0, -6.015) normal (0, 0, 1) x (1, 0, 0) in component "R_F_Wheel_Base"
  line L0 (7, -47.65) -> (7, -39.65)
  line L1 (7, -39.65) -> (-9.5, -57.351)
  line L2 (-9.5, -57.351) -> (-9.5, -72.351)
  line L3 (-9.5, -72.351) -> (5.5, -72.351)
  line L4 (5.5, -72.351) -> (5.5, -57.351)
  line L5 (5.5, -57.351) -> (7, -47.65)
  line L6 (5.5, -57.351) -> (-9.5, -57.351)
  constraint coincident L4.end L5.start
  constraint coincident L1.end L2.start
extrude "Extrude4''''''''''" cut sketch "Sketch4 (11)" against normal blind 2 contours L0 L1 L5 L6 bodies 22 in component "R_F_Wheel_Base"
fillet "Fillet1'''''" radius 11.5 1 edges at (7, -47.65, -17.015) on bodies 22 in component "R_F_Wheel_Base"
fillet "Fillet2''''''" radius 14 1 edges at (16, -47.65, -17.015) on bodies 22 in component "R_F_Wheel_Base"
sketch "Sketch5 (8)" plane through (0, 0, -26.015) normal (0, 0, -1) x (-1, 0, 0) in component "R_F_Wheel_Base"
  arc A0 (-16, -38.3973) -> (-10.1604, -49.7731) centre (-2, -38.3973) ccw
  arc A1 (-5.5, -57.351) -> (-10.1604, -49.7731) centre (-16.8635, -59.1175) ccw
  line L0 (-5.5, -57.351) -> (-5.5, -72.351)
  line L1 (-5.5, -72.351) -> (9.5, -72.351)
  line L2 (9.5, -72.351) -> (9.5, -57.351)
  line L3 (9.5, -57.351) -> (-7, -39.65)
  line L4 (-7, -39.65) -> (-7, -31.65)
  line L5 (-7, -31.65) -> (-16, -31.65)
  line L6 (-16, -31.65) -> (-16, -38.3973)
  line L7 (9.5, -57.351) -> (-5.5, -57.351)
  constraint coincident L2.end L3.start
  constraint coincident A1.start L0.start
extrude "Extrude5'''''''" add sketch "Sketch5 (8)" along normal blind 2 contours L0 L1 L2 L7 bodies 22 in component "R_F_Wheel_Base"
extrude "Extrude6'''''''" cut 1 faces at (0.5, -67.351, -6.015) along direction (0, 0, -1) blind 2 on bodies 22 bodies 22 in component "R_F_Wheel_Base"
sketch "Sketch6 (8)" plane through (0, -26.65, 0) normal (0, 1, 0) x (-1, 0, 0) in component "R_F_Wheel_Base"
  circle A0 centre (-11.5, -4.1) radius 1
  circle A1 centre (-11.5, -29.93) radius 1
  line L0 (-5.5, -29.015) -> (-5.5, -5.015)
  line L1 (-5.5, -5.015) -> (-7.1, -5.015)
  line L2 (-7.1, -5.015) -> (-7.1, -0.5642)
  line L3 (-7.1, -0.5642) -> (-15.9, -0.5642)
  line L4 (-15.9, -0.5642) -> (-15.9, -5.015)
  line L5 (-15.9, -5.015) -> (-17.5, -5.015)
  line L6 (-17.5, -5.015) -> (-17.5, -29.015)
  line L7 (-17.5, -29.015) -> (-15.9, -29.015)
  line L8 (-15.9, -29.015) -> (-15.9, -33.466)
  line L9 (-15.9, -33.466) -> (-7.1, -33.466)
  line L10 (-7.1, -33.466) -> (-7.1, -29.015)
  line L11 (-7.1, -29.015) -> (-5.5, -29.015)
  line L12 (-16, -27.03) -> (-7, -27.03)
  line L13 (-16, -7) -> (-16, -27.03)
  line L14 (-7, -27.03) -> (-7, -7)
  line L15 (-7, -27.03) -> (-16, -27.03)
  line L16 (-16, -27.03) -> (-16, -7)
  line L17 (-16, -7) -> (-7, -7)
  line L18 (-7, -7) -> (-7, -27.03)
  line L19 (-15.91, -7.09) -> (-7.09, -7.09)
  line L20 (-7.09, -7.09) -> (-7.09, -26.94)
  line L21 (-7.09, -26.94) -> (-15.91, -26.94)
  line L22 (-15.91, -26.94) -> (-15.91, -7.09)
  dimension "d553" = 0.09
  constraint horizontal L15
  constraint vertical L16
  constraint horizontal L17
  constraint vertical L18
  constraint coincident L13.start L16.end
  constraint coincident L12.end L14.start
extrude "Extrude7''''" add sketch "Sketch6 (8)" along normal blind 3 contours L19 L20 L21 L22 bodies 22 in component "R_F_Wheel_Base"
sketch "Sketch7 (6)" plane through (0, 0, -8.015) normal (0, 0, 1) x (1, 0, 0) in component "R_F_Wheel_Base"
  arc A0 (10.1604, -49.7731) -> (16, -38.3973) centre (2, -38.3973) ccw
  line L0 (16, -38.3973) -> (16, -31.65)
  line L1 (16, -31.65) -> (7, -31.65)
  line L2 (7, -31.65) -> (7, -39.65)
  line L3 (7, -39.65) -> (-9.5, -57.351)
  line L4 (-9.5, -57.351) -> (-9.5, -72.351)
  line L5 (-9.5, -72.351) -> (5.5, -72.351)
  line L6 (5.5, -72.351) -> (5.5, -57.351)
  arc A1 (10.1604, -49.7731) -> (5.5, -57.351) centre (16.8635, -59.1175) ccw
  line L7 (-9.5, -57.351) -> (5.5, -57.351)
  circle A2 centre (-2, -64.851) radius 2
  line L8 (-2, -64.851) -> (-6.572, -64.851) construction
  line L9 (-2, -64.851) -> (2.572, -64.851) construction
  circle A3 centre (-6.572, -64.851) radius 0.75
  circle A4 centre (2.572, -64.851) radius 0.75
  dimension "d556" = 4
  dimension "d557" = 4.572
  dimension "d558" = 4.572
  dimension "d559" = 1.5
  dimension "d560" = 1.5
  constraint coincident L3.end L4.start
  constraint coincident L6.end A1.end
  constraint coincident A2.centre L8.start
  constraint horizontal L8
  constraint parallel L8 L9
  constraint coincident L8.end A3.centre
  constraint coincident L9.end A4.centre
  measures "d556" diameter of A2
  measures "d557" distance of A2.centre L8.end
  measures "d558" distance of A2.centre L9.end
  measures "d559" diameter of A3
  measures "d560" diameter of A4
extrude "Extrude8''''" cut sketch "Sketch7 (6)" against normal blind 20 contours A2 | A3 | A4 bodies 22 in component "R_F_Wheel_Base"
sketch "Sketch8 (3)" plane through (0, 0, -28.015) normal (0, 0, -1) x (-1, 0, 0) in component "R_F_Wheel_Base"
  circle A0 centre (2, -64.851) radius 2
  circle A1 centre (6.572, -64.851) radius 0.75
  circle A2 centre (-2.572, -64.851) radius 0.75
  line L0 (9.5, -57.351) -> (-5.5, -57.351)
  line L1 (-5.5, -57.351) -> (-5.5, -72.351)
  line L2 (-5.5, -72.351) -> (9.5, -72.351)
  line L3 (9.5, -72.351) -> (9.5, -57.351)
  line L4 (8.1, -69.951) -> (-4.1, -69.951)
  line L5 (-4.1, -69.951) -> (-4.1, -59.751)
  line L6 (-4.1, -59.751) -> (8.1, -59.751)
  line L7 (8.1, -59.751) -> (8.1, -69.951)
  line L8 (8.1, -69.951) -> (-4.1, -59.751) construction
  line L9 (-4.1, -69.951) -> (8.1, -59.751) construction
  point P0 (2, -64.851)
  dimension "d563" = 12.2
  dimension "d564" = 10.2
  constraint horizontal L4
  constraint perpendicular L4 L5
  constraint parallel L4 L6
  constraint parallel L5 L7
  constraint coincident L8 P0
  constraint coincident L9 P0
  constraint coincident P0 A0.centre
  measures "d563" distance of L5.end L6.end
  measures "d564" distance of L4.end L5.end
extrude "Extrude9'''" cut sketch "Sketch8 (3)" against normal blind 18.841 contours L4 L5 L6 L7 bodies 22 in component "R_F_Wheel_Base"
sketch "Sketch1 (13)" plane through (0, -26.65, 0) normal (0, -1, 0) x (1, 0, 0) in component "L_F_Wheel_Base"
  line L0 (0, -40) -> (-5, -45)
  line L1 (-5, -45) -> (-5, -79.85)
  line L2 (-5, -79.85) -> (0, -84.85)
  line L3 (0, -84.85) -> (0, -97)
  arc A0 (0, -97) -> (3, -100) centre (3, -97) ccw
  line L4 (3, -100) -> (6, -103)
  line L5 (6, -103) -> (25, -103)
  line L6 (25, -103) -> (28, -100)
  line L7 (28, -100) -> (154, -100)
  arc A1 (154, -100) -> (157, -97) centre (154, -97) ccw
  line L8 (157, -97) -> (157, -94)
  arc A2 (160, -91) -> (157, -94) centre (160, -94) ccw
  line L9 (160, -91) -> (181.27, -91)
  arc A3 (181.27, -91) -> (184.27, -88) centre (181.27, -88) ccw
  line L10 (184.27, -88) -> (184.27, -12)
  arc A4 (184.27, -12) -> (181.27, -9) centre (181.27, -12) ccw
  line L11 (181.27, -9) -> (160, -9)
  arc A5 (157, -6) -> (160, -9) centre (160, -6) ccw
  line L12 (157, -6) -> (157, -3)
  arc A6 (157, -3) -> (154, 0) centre (154, -3) ccw
  line L13 (154, 0) -> (28, 0)
  line L14 (28, 0) -> (25, 3)
  line L15 (25, 3) -> (6, 3)
  line L16 (6, 3) -> (3, 0)
  arc A7 (3, 0) -> (0, -3) centre (3, -3) ccw
  line L17 (0, -3) -> (0, -40)
  circle A8 centre (3, -97) radius 1.0625
  circle A9 centre (3, -71) radius 1.0625
  circle A10 centre (22, -71) radius 1.0625
  circle A11 centre (3, -29) radius 1.0625
  circle A12 centre (3, -3) radius 1.0625
  circle A13 centre (22, -29) radius 1.0625
  circle A14 centre (90, -16) radius 1.0625
  circle A15 centre (114, -16) radius 1.0625
  circle A16 centre (90, -30.28) radius 1.0625
  circle A17 centre (114, -30.28) radius 1.0625
  circle A18 centre (114, -69.72) radius 1.0625
  circle A19 centre (90, -84) radius 1.0625
  circle A20 centre (90, -69.72) radius 1.0625
  circle A21 centre (114, -84) radius 1.0625
  line L18 (92.5, -27.97) -> (92.5, -18.97)
  line L19 (92.5, -18.97) -> (112.5, -18.97)
  line L20 (112.5, -18.97) -> (112.5, -27.97)
  line L21 (112.5, -27.97) -> (92.5, -27.97)
  circle A22 centre (11.5, -70.07) radius 1
  circle A23 centre (11.5, -4.1) radius 1
  circle A24 centre (11.5, -29.93) radius 1
  line L22 (92.5, -81.36) -> (92.5, -72.36)
  line L23 (92.5, -72.36) -> (112.5, -72.36)
  line L24 (112.5, -72.36) -> (112.5, -81.36)
  line L25 (112.5, -81.36) -> (92.5, -81.36)
  circle A25 centre (89.585, -23.47) radius 1
  circle A26 centre (115.415, -76.86) radius 1
  line L26 (16, -72.97) -> (16, -93)
  line L27 (16, -93) -> (7, -93)
  line L28 (7, -93) -> (7, -72.97)
  line L29 (7, -72.97) -> (16, -72.97)
  line L30 (16, -7) -> (16, -27.03)
  line L31 (16, -27.03) -> (7, -27.03)
  line L32 (7, -27.03) -> (7, -7)
  line L33 (7, -7) -> (16, -7)
  circle A27 centre (11.5, -95.9) radius 1
  circle A28 centre (89.585, -76.86) radius 1
  circle A29 centre (115.415, -23.47) radius 1
  line L34 (127.5, -73.5) -> (124.5, -73.5)
  line L35 (124.5, -73.5) -> (124.5, -68.5)
  line L36 (124.5, -68.5) -> (127.5, -68.5)
  line L37 (127.5, -68.5) -> (127.5, -73.5)
  line L38 (183.5, -73.5) -> (180.5, -73.5)
  line L39 (180.5, -73.5) -> (180.5, -68.5)
  line L40 (180.5, -68.5) -> (183.5, -68.5)
  line L41 (183.5, -68.5) -> (183.5, -73.5)
  line L42 (127.5, -31.5) -> (124.5, -31.5)
  line L43 (124.5, -31.5) -> (124.5, -26.5)
  line L44 (124.5, -26.5) -> (127.5, -26.5)
  line L45 (127.5, -26.5) -> (127.5, -31.5)
  line L46 (183.5, -31.5) -> (180.5, -31.5)
  line L47 (180.5, -31.5) -> (180.5, -26.5)
  line L48 (180.5, -26.5) -> (183.5, -26.5)
  line L49 (183.5, -26.5) -> (183.5, -31.5)
  line L50 (36.83, -3.81) -> (36.83, -13.97)
  line L51 (36.83, -13.97) -> (19.05, -13.97)
  line L52 (19.05, -13.97) -> (19.05, -3.81)
  line L53 (19.05, -3.81) -> (36.83, -3.81)
  line L54 (36.83, -96.52) -> (19.05, -96.52)
  line L55 (19.05, -96.52) -> (19.05, -86.36)
  line L56 (19.05, -86.36) -> (36.83, -86.36)
  line L57 (36.83, -86.36) -> (36.83, -96.52)
  line L58 (114.3, -3.81) -> (130.81, -3.81)
  line L59 (130.81, -3.81) -> (130.81, -13.97)
  line L60 (130.81, -13.97) -> (114.3, -13.97)
  line L61 (114.3, -13.97) -> (114.3, -3.81)
  line L62 (114.3, -96.52) -> (114.3, -86.36)
  line L63 (114.3, -86.36) -> (130.81, -86.36)
  line L64 (130.81, -86.36) -> (130.81, -96.52)
  line L65 (130.81, -96.52) -> (114.3, -96.52)
  line L66 (5.5, -5.015) -> (5.5, -29.015)
  line L67 (17.5, -29.015) -> (17.5, -5.015)
  line L68 (17.5, -5.015) -> (5.5, -29.015) construction
  line L69 (5.5, -5.015) -> (17.5, -29.015) construction
  line L70 (7, -3) -> (7, -5.015) construction
  line L71 (16, -3) -> (16, -5.015) construction
  line L72 (7.1, -3) -> (7.1, -5.015) construction
  line L73 (15.9, -3) -> (15.9, -5.015) construction
  line L74 (5.5, -5.015) -> (7.1, -5.015)
  line L75 (17.5, -5.015) -> (15.9, -5.015)
  line L76 (15.9, -5.015) -> (15.9, -0.5642)
  line L77 (15.9, -0.5642) -> (7.1, -0.5642)
  line L78 (7.1, -0.5642) -> (7.1, -5.015)
  line L79 (5.5, -29.015) -> (7.1, -29.015)
  line L80 (17.5, -29.015) -> (15.9, -29.015)
  line L81 (7.1, -29.015) -> (7.1, -33.466)
  line L82 (7.1, -33.466) -> (15.9, -33.466)
  line L83 (15.9, -33.466) -> (15.9, -29.015)
  point P0 (11.5, -17.015)
  dimension "d517_1" = 12
  dimension "d518_1" = 24
  dimension "d519_1" = -0.1
  dimension "d520_1" = 0.1
  dimension "d521_1" = 1.6
  dimension "d522_1" = 4.4508
  dimension "d523_1" = 8.8
  dimension "d524_1" = 4.4508
  dimension "d525_1" = 1.6
  dimension "d526_1" = 3.5642
  dimension "d527_1" = 5.5
  dimension "d528_1" = 1.55
  dimension "d529_1" = 1.6
  dimension "d530_1" = 1.6
  dimension "d531_1" = 4.451
  dimension "d532_1" = 7.1
  dimension "d533_1" = 4.451
  dimension "d534_1" = 32.9018
  constraint parallel L66 L67
  constraint coincident L68 P0
  constraint coincident L69 P0
  constraint perpendicular L72 L74
  constraint perpendicular L73 L75
  constraint vertical L76
  constraint horizontal L77
  constraint vertical L78
  constraint perpendicular L17 L79
  constraint perpendicular L67 L80
  constraint vertical L81
  constraint horizontal L82
  constraint vertical L83
  measures "d517_1" distance of L66.end L67.start
  measures "d518_1" distance of L66.start L66.end
  measures "d521_1" distance of L67.end L73.end
  measures "d522_1" distance of L73.end L76.end
  measures "d523_1" distance of L76.end L77.end
  measures "d524_1" distance of L72.end L77.end
  measures "d525_1" distance of L66.start L72.end
  measures "d526_1" distance of L15 L77
  measures "d527_1" distance of L17 L66
  measures "d528_1" distance of L52 L67
  measures "d529_1" distance of L66.end L79.end
  measures "d530_1" distance of L67.start L80.end
  measures "d531_1" distance of L80.end L82.end
  measures "d532_1" distance of L17 L81
  measures "d533_1" distance of L79 L82
  measures "d534_1" distance of L77 L82
extrude "Extrude1'''''''''''''''" add sketch "Sketch1 (13)" along normal blind 5 separate body contours L30 L31 L32 L33 | L66 L67 L74 L75 L76 L77 L78 L79 L80 L81 L82 L83 makes body 23 in component "L_F_Wheel_Base"
sketch "Sketch2 (14)" plane through (0, -31.65, 0) normal (0, -1, 0) x (1, 0, 0) in component "L_F_Wheel_Base"
  circle A0 centre (11.5, -4.1) radius 1
  circle A1 centre (11.5, -29.93) radius 1
  line L0 (5.5, -5.015) -> (5.5, -29.015)
  line L1 (5.5, -29.015) -> (7.1, -29.015)
  line L2 (7.1, -29.015) -> (7.1, -33.466)
  line L3 (7.1, -33.466) -> (15.9, -33.466)
  line L4 (15.9, -33.466) -> (15.9, -29.015)
  line L5 (15.9, -29.015) -> (17.5, -29.015)
  line L6 (17.5, -29.015) -> (17.5, -5.015)
  line L7 (17.5, -5.015) -> (15.9, -5.015)
  line L8 (15.9, -5.015) -> (15.9, -0.5642)
  line L9 (15.9, -0.5642) -> (7.1, -0.5642)
  line L10 (7.1, -0.5642) -> (7.1, -5.015)
  line L11 (7.1, -5.015) -> (5.5, -5.015)
  line L12 (16, -26.015) -> (7, -26.015)
  line L13 (7, -26.015) -> (7, -8.015)
  line L14 (7, -8.015) -> (16, -8.015)
  line L15 (16, -8.015) -> (16, -26.015)
  line L16 (16, -26.015) -> (7, -8.015) construction
  line L17 (7, -26.015) -> (16, -8.015) construction
  point P0 (11.5, -17.015)
  dimension "d537_1" = 18
  constraint horizontal L12
  constraint perpendicular L12 L13
  constraint parallel L12 L14
  constraint parallel L13 L15
  constraint coincident L16 P0
  constraint coincident L17 P0
  measures "d537_1" distance of L12.end L13.end
extrude "Extrude2'''''''''''''" add sketch "Sketch2 (14)" along normal blind 16 contours L12 L13 L14 L15 bodies 23 in component "L_F_Wheel_Base"
sketch "Sketch3 (10)" plane through (0, 0, -26.015) normal (0, 0, -1) x (-1, 0, 0) in component "L_F_Wheel_Base"
  line L0 (-7, -31.65) -> (-16, -31.65)
  line L1 (-16, -31.65) -> (-16, -47.65)
  line L2 (-16, -47.65) -> (-7, -47.65)
  line L3 (-7, -47.65) -> (-7, -31.65)
  line L4 (-16, -39.65) -> (-7, -47.65)
  line L5 (-16, -31.65) -> (-7, -39.65)
  line L6 (-16, -47.65) -> (-16, -72.351) construction
  line L7 (-16, -72.351) -> (35, -72.351) construction
  line L8 (9.5, -72.351) -> (-5.5, -72.351)
  line L9 (-5.5, -72.351) -> (-5.5, -57.351)
  line L10 (9.5, -57.351) -> (9.5, -72.351)
  line L11 (9.5, -57.351) -> (1.25, -48.5005)
  line L12 (-7, -39.65) -> (1.25, -48.5005)
  line L13 (-7, -47.65) -> (-5.5, -57.351)
  dimension "d540_1" = 24.701
  dimension "d541_1" = 15
  dimension "d542_1" = 15
  constraint midpoint L1 L4.start
  constraint coincident L2.end L3.start
  constraint coincident L0.end L1.start
  constraint midpoint L3 L5.end
  constraint coincident L1.end L2.start
  constraint perpendicular L2 L6
  constraint perpendicular L6 L7
  constraint horizontal L8
  constraint vertical L9
  constraint vertical L10
  constraint midpoint L7 L8.start
  constraint parallel L11 L12
  measures "d540_1" distance of L1.end L6.end
  measures "d541_1" distance of L8.start L8.end
  measures "d542_1" distance of L8.start L10.start
extrude "Extrude3'''''''''''" add sketch "Sketch3 (10)" against normal blind 20 contours L3 L8 L9 L10 L11 L12 L13 bodies 23 in component "L_F_Wheel_Base"
sketch "Sketch4 (12)" plane through (0, 0, -6.015) normal (0, 0, 1) x (1, 0, 0) in component "L_F_Wheel_Base"
  line L0 (7, -47.65) -> (7, -39.65)
  line L1 (7, -39.65) -> (-9.5, -57.351)
  line L2 (-9.5, -57.351) -> (-9.5, -72.351)
  line L3 (-9.5, -72.351) -> (5.5, -72.351)
  line L4 (5.5, -72.351) -> (5.5, -57.351)
  line L5 (5.5, -57.351) -> (7, -47.65)
  line L6 (5.5, -57.351) -> (-9.5, -57.351)
  constraint coincident L4.end L5.start
  constraint coincident L1.end L2.start
extrude "Extrude4'''''''''''" cut sketch "Sketch4 (12)" against normal blind 2 contours L0 L1 L5 L6 bodies 23 in component "L_F_Wheel_Base"